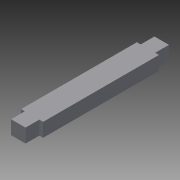
# Autodesk Inventor part: Stopper
Saved by Autodesk Inventor 2015 SP1 (Build 190203100, 203)
## iProperties
Created: 2014-08-09
Part Number: Stopper
Material: Generic
Document SubType Name: Modeling
Designer: Patrick Camilleri
Density: 1 g/cm^3
Appearance: Default
Author: Patrick Camilleri
Autodesk Inventor part; units mm, degrees
ref_plane "YZ Plane" through (0, 0, 0) normal (1, 0, 0) x (0, 1, 0)
ref_plane "XZ Plane" through (0, 0, 0) normal (0, 1, 0) x (-1, 0, 0)
ref_plane "XY Plane" through (0, 0, 0) normal (0, 0, 1) x (1, 0, 0)
sketch "Sketch1" plane through (0, 0, 0) normal (0, 0, 1) x (1, 0, 0)
  line L0 (-4, 21) -> (4, 21)
  line L1 (4, 21) -> (4, -21)
  line L2 (4, -21) -> (-4, -21)
  line L3 (-4, -21) -> (-4, 21)
  line L4 (-4, 21) -> (4, -21) construction
  line L5 (4, 21) -> (-4, -21) construction
  point P0 (0, 0)
  dimension "d0" = 8
  dimension "d1" = 42
  constraints: 12 end point, 2 midpoint, 2 parallel, 1 horizontal, 1 perpendicular
  measures "d0" distance of L1.end L2.end
  measures "d1" distance of L0.end L1.end
extrude "Extrusion1" add sketch "Sketch1" along normal blind 5
sketch "Sketch2" plane through (0, 0, 5) normal (0, 0, 1) x (1, 0, 0)
  line L0 (4, 21) -> (-4, 21) projected
  line L1 (-2.625, 26) -> (2.625, 26)
  line L2 (2.625, 26) -> (2.625, 21)
  line L3 (2.625, 21) -> (-2.625, 21)
  line L4 (-2.625, 21) -> (-2.625, 26)
  line L5 (-2.625, 26) -> (2.625, 21) construction
  line L6 (2.625, 26) -> (-2.625, 21) construction
  point P0 (0, 0)
  point P1 (0, 23.5)
  point P2 (0, 21)
  dimension "d4" = 5.25
  dimension "d5" = 5
  constraints: 12 end point, 4 midpoint, 2 parallel, 1 horizontal, 1 perpendicular
  measures "d4" distance of L2.end L3.end
  measures "d5" distance of L1.end L2.end
extrude "Extrusion2" add sketch "Sketch2" against normal blind 5
mirror "Mirror1" about plane through (0, 0, 0) normal (0, 1, 0) of "Extrusion2"
equation "\"kerf\" = 0.15"
body "Solid1"
